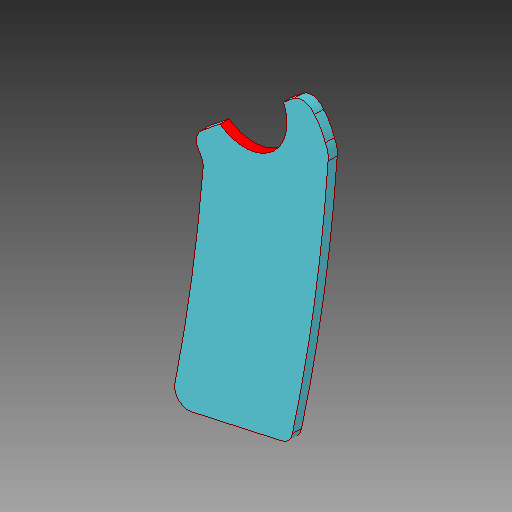
# Autodesk Inventor part: brazocuadrado
Saved by Autodesk Inventor 2019 (Build 230136000, 136)
## iProperties
Part Number: brazocuadrado
Material: Genérico
Document SubType Name: Chapa
Designer: Kevin
Density: 1 g/cm^3
Sheet Metal Rule: Por defecto_mm
Appearance: Valor por defecto
Author: Kevin
Autodesk Inventor part; units mm, degrees
ref_plane "YZ Plane" through (0, 0, 0) normal (1, 0, 0) x (0, 1, 0)
ref_plane "Plano de trabajo14" through (0, 0, 40) normal (0, 0, 1) x (1, 0, 0)
sketch "Boceto6" plane through (0, 0, 40) normal (0, 0, 1) x (1, 0, 0)
  line L0 (49.7736, 62.508) -> (29.5128, 46.2994)
  line L1 (28.7888, 42.4568) -> (29.4835, 41.2536)
  line L2 (47.1158, -3.8365) -> (27.2606, -8.2224)
  arc A0 (29.5128, 46.2994) -> (28.7888, 42.4568) centre (31.3869, 43.9568) ccw
  arc A1 (29.8562, 39.3361) -> (29.4835, 41.2536) centre (26.8854, 39.7536) ccw
  arc A2 (54.2458, 61.6654) -> (49.7736, 62.508) centre (51.6477, 60.1654) ccw
  arc A3 (23.6427, -4.8755) -> (27.2606, -8.2224) centre (26.6135, -5.293) ccw
  arc A4 (47.1158, -3.8365) -> (49.4395, -1.3246) centre (46.4687, -0.9071) ccw
  arc A5 (57.2604, 54.324) -> (56.6392, 57.5198) centre (52.3091, 55.0198) ccw
  arc A6 (56.6392, 57.5198) -> (54.2458, 61.6654) centre (47.0339, 54.7379) ccw
  arc A7 (49.4395, -1.3246) -> (57.2604, 54.324) centre (-341.7788, 82.0314) ccw
  arc A8 (23.6427, -4.8755) -> (29.8562, 39.3361) centre (-368.7404, 72.8128) ccw
  line L3 (51.5494, 60.0868) -> (31.3869, 43.9568)
  line L4 (31.3869, 43.9568) -> (32.0816, 42.7536)
  arc A9 (32.8399, 39.0157) -> (32.0816, 42.7536) centre (26.8854, 39.7536) ccw
  arc A10 (26.6185, -5.2919) -> (32.8399, 39.0157) centre (-368.7404, 72.8128) ccw
  line L5 (26.6185, -5.2919) -> (46.4607, -0.9089)
  arc A11 (46.4607, -0.9089) -> (54.2765, 54.6606) centre (-341.7788, 82.0314) ccw
  arc A12 (54.2765, 54.6606) -> (53.8619, 56.2803) centre (52.3091, 55.0198) ccw
  arc A13 (53.8619, 56.2803) -> (51.5494, 60.0868) centre (47.0339, 54.7379) ccw
  dimension "d106" = 3
  constraints: 28 point on circle, 14 centre point, 12 end point, 6 tangent, 3 equal radius, 7 other
  measures "d106" distance between parallel lines of L0 L3
extrude "Extrusión11" add sketch "Boceto6" against normal blind 2 contours A2 A6 A5 A7 A4 L2 A3 A8 A1 L1 A0 L0 | A13 A12 A11 L5 A10 A9 L4 L3
ref_plane "Plano de trabajo15" through (0, 0, 40) normal (0, 0, -1) x (-1, 0, 0)
sketch "Boceto34" plane through (0, 0, 40) normal (0, 0, 1) x (1, 0, 0)
  line L0 (47.4839, 60.6763) -> (33.5541, 49.5324)
  line L1 (39.6432, 54.4037) -> (42.1142, 54.4037) construction
  line L2 (39.6432, 54.4037) -> (42.3572, 54.4037) construction
  arc A0 (33.5541, 49.5324) -> (47.4839, 60.6763) centre (38.9752, 57.0342) ccw
  point P0 (0, 0)
  dimension "d154" = 18.511
  constraints: 6 end point, 2 horizontal, 2 point on circle, 1 centre point, 1 point on line
  measures "d154" diameter of A0
extrude "Extrusión26" cut sketch "Boceto34" against normal blind 10
equation "\"Radio_pliegue\" = Grosor"
equation "\"Anchura_desahogo_plegado\" = Grosor"
equation "\"Profundidad_desahogo_plegado\" = 0.5 * Grosor"
equation "\"Tamaño_destalonado\" = 4 * Grosor"
equation "\"Remanente_mínimo\" = 2 * Grosor"
equation "\"Radiodetransición\" = Radio_pliegue"
equation "\"Tamaño_de_radio_de_Jacobi\" = Radio_pliegue"
equation "\"TamañoSeparación\" = Grosor"
equation "\"Grosor\" = 0.5"
